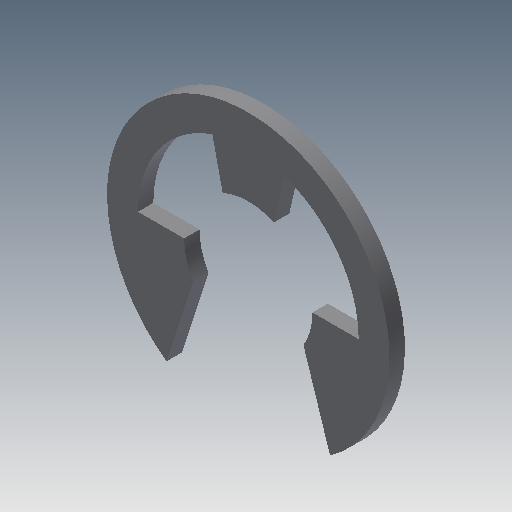
# Autodesk Inventor part: NETW5
Saved by Autodesk Inventor 2019.4 (Build 234330000, 330)
## iProperties
Category: PARTsolutions
Company: MISUMI
Created: 2019-06-15
Part Number: NETW5
Material: 一般
Catalog Web Link: www.cadenas.de
Description: NETW, NETWS-Retaining Rings - E
Vendor: MISUMI
Document SubType Name: Modeling
Designer: psadmin
Manufacturer: MISUMI
Mass: 0.0256836 g
Surface Area: 1.19896 cm^2
Volume: 0.0256836 cm^3
Density: 1 g/cm^3
Appearance: PSOLRGB-175-175-175
PSOL_IDENT_0: {$CADENAS_DATA\23d-libs\misumi\metric\28_keys_magnets\netw.prj},158 {VTYP=3D},{NB=NETW5},{LINA=NETW5
PSOL_IDENT_1: },{NN=NETW, NETWS},{DATE=30.03.2018 06:58:56},{GEOMDATE=11.08.2011 06:04:00},{VERSION=},{LINEID=70},
PSOL_IDENT_2: {WBVAR=MAT},{WBNUMERIC=}  {NB=NETW5},{LINA=NETW5},{KT=DUMMY},{PN=NETW5},{TS=NETW},{MAT=},{HARD=44~53
PSOL_IDENT_3: HRC},{ST=Trivalent Chromate},{NO=5},{DD=5.0},{DDTOL=0/-0.12},{D=11},{DTOL=+0.2/-0.2},{H=4.3},{HTOL=0
PSOL_IDENT_4: /-0.30},{TT=0.6},{TTTOL=+0.4/-0.4},{DD1=6~},{LESS=~8},{DD2=5.0},{DD2TOL=+0.075/0},{MM=0.7},{MMTOL=+0
PSOL_IDENT_5: .1/0},{NN=1.2},{MATRR=Steel for Springs},{D1=8.600},{H1=2.800},{DEG1=25.400},{DEG2=35.700}
NN: 1.2
NT: Retaining Rings - E
NB: NETW5
NBSYN: $PN.
LINA: NETW5
PN: NETW5
MAT: Steel for Springs
HARD: 44~53HRC
ST: Trivalent Chromate
NO: 5
DD: 5
DDTOL: 0/-0.12
D: 11
DTOL: +0.2/-0.2
H: 4.3
HTOL: 0/-0.30
TT: 0.6
TTTOL: +0.4/-0.4
DD1: 6~
LESS: ~8
DD2: 5
DD2TOL: +0.075/0
MM: 0.7
MMTOL: +0.1/0
D1: 8.6
H1: 2.8
DEG1: 25.4
DEG2: 35.7
SUPPLIER: MISUMI
ARTICLENO: NETW5
BOMINFO: NETW5
CREATOR: CADENAS GmbH
Title: NETW5
Author: Cadenas PARTsolutions
Comments: Retaining Rings - E
Autodesk Inventor part; units mm, degrees
sketch "Sketch_1" plane through (0, 0, 0) normal (0, 0, 1) x (1, 0, 0)
  arc A0 (3.1835, -4.485) -> (-3.1835, -4.485) centre (0, 0) ccw
  line L0 (-3.1835, -4.485) -> (-2.15, -1.2757)
  arc A1 (-2.5, 0) -> (-2.15, -1.2757) centre (0, 0) ccw
  line L1 (-2.5, 0) -> (-4.3, 0)
  arc A2 (-1.4, 4.0657) -> (-4.3, 0) centre (0, 0) ccw
  line L2 (-1.4, 4.0657) -> (-1.0001, 2.2912)
  arc A3 (1.0001, 2.2912) -> (-1.0001, 2.2912) centre (0, 0) ccw
  line L3 (1.0001, 2.2912) -> (1.4, 4.0657)
  arc A4 (4.3, 0) -> (1.4, 4.0657) centre (0, 0) ccw
  line L4 (4.3, 0) -> (2.5, 0)
  arc A5 (2.15, -1.2757) -> (2.5, 0) centre (0, 0) ccw
  line L5 (2.15, -1.2757) -> (3.1835, -4.485)
  constraints: 12 end point, 12 point on circle, 6 centre point
extrude "Extrusion1" add sketch "Sketch_1" along normal mid plane 0.6
ref_plane "COMBINATION_MODULE_XY" through (0, 0, 0.3) normal (0, 0, 1) x (1, 0, 0)
ref_plane "COMBINATION_MODULE_YZ" through (0, 0, 0.3) normal (1, 0, 0) x (0, 1, 0)
ref_plane "COMBINATION_MODULE_ZX" through (0, 0, 0.3) normal (0, 1, 0) x (0, 0, 1)
ref_plane "ring_to_screw_XY" through (0, 0, 0) normal (0, 0, 1) x (1, 0, 0)
ref_plane "ring_to_screw_YZ" through (0, 0, 0) normal (1, 0, 0) x (0, 1, 0)
ref_plane "ring_to_screw_ZX" through (0, 0, 0) normal (0, 1, 0) x (0, 0, 1)
body "Solid1"
